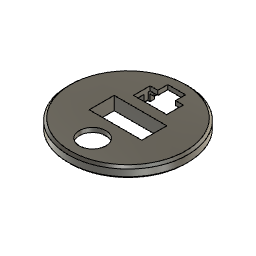
PowerBank RedBull (Autodesk Fusion 360 design; units mm, degrees)
Autodesk Fusion 360 part; units mm, degrees
sketch "Boceto1" plane through (0, 0, 0) normal (0, 0, 1) x (1, 0, 0)
  circle A0 centre (0, 0) radius 27
  dimension "d1" = 54
  constraint coincident A0.centre origin
  measures "d1" diameter of A0
extrude "Extruir1" add sketch "Boceto1" along normal blind 5
sketch "Boceto2" plane through (0, 0, 0) normal (0, 0, -1) x (1, 0, 0)
  circle A0 centre (0, 0) radius 27
  circle A1 centre (0, 0) radius 26
  dimension "d6" = 52
  constraint coincident A0.centre A1.centre
  measures "d6" diameter of A1
extrude "Extruir2" cut sketch "Boceto2" against normal blind 3 contours A1
sketch "Boceto3" plane through (0, 0, 5) normal (0, 0, 1) x (-1, 0, 0)
  circle A0 centre (0, 0) radius 27
  line L0 (-11.4, 5.15) -> (11.4, 5.15)
  line L1 (11.4, 5.15) -> (11.4, -5.15)
  line L2 (11.4, -5.15) -> (-11.4, -5.15)
  line L3 (-11.4, -5.15) -> (-11.4, 5.15)
  line L4 (-11.4, 5.15) -> (11.4, -5.15) construction
  line L5 (11.4, 5.15) -> (-11.4, -5.15) construction
  line L6 (0, -27) -> (0, 27) construction
  line L7 (0, 5.15) -> (0, 16) construction
  circle A1 centre (0, 16) radius 6
  dimension "d9" = 10.3
  dimension "d10" = 22.8
  dimension "d11" = 12
  constraint horizontal L0
  constraint perpendicular L0 L1
  constraint parallel L0 L2
  constraint parallel L1 L3
  constraint coincident L4 A0.centre
  constraint coincident L5 A0.centre
  constraint coincident A0.centre origin
  constraint coincident A0 L6.start
  constraint coincident A0 L6.end
  constraint perpendicular L0 L6
  constraint midpoint L0 L7.start
  constraint coincident L6 L7.end
  constraint perpendicular L0 L7
  constraint coincident L7.end A1.centre
  measures "d9" distance of L0.start L2.end
  measures "d10" distance of L0.start L0.end
  measures "d11" diameter of A1
extrude "Extruir3" cut sketch "Boceto3" against normal blind 3 contours L0 L1 L2 L3 | A1
sketch "Boceto4" plane through (0, 0, 3) normal (0, 0, -1) x (1, 0, 0)
  circle A0 centre (0, 16) radius 6
  line L0 (-11.4, -5.15) -> (-11.4, 5.15)
  line L1 (-11.4, 5.15) -> (11.4, 5.15)
  line L2 (11.4, 5.15) -> (11.4, -5.15)
  line L3 (11.4, -5.15) -> (-11.4, -5.15)
  circle A1 centre (0, 0) radius 26
  line L4 (-12.4, 6.15) -> (12.4, 6.15)
  line L5 (12.4, 6.15) -> (12.4, -6.15)
  line L6 (12.4, -6.15) -> (-12.4, -6.15)
  line L7 (-12.4, -6.15) -> (-12.4, 6.15)
  line L8 (-12.4, 6.15) -> (12.4, -6.15) construction
  line L9 (12.4, 6.15) -> (-12.4, -6.15) construction
  dimension "d14" = 24.8
  dimension "d15" = 12.3
  constraint horizontal L4
  constraint perpendicular L4 L5
  constraint parallel L4 L6
  constraint parallel L5 L7
  constraint coincident L8 A1.centre
  constraint coincident L9 A1.centre
  constraint coincident A1.centre origin
  measures "d14" distance of L5.end L6.end
  measures "d15" distance of L4.end L5.end
extrude "Extruir4" add sketch "Boceto4" along normal blind 4 contours L4 L5 L6 L7
chamfer "Chaflán1" distance 1 angle 45 1 edges at (-25.1728, -9.7636, 5)
extrude "Extruir5" add 1 faces at (12.4, -2.05, 0.3333) along direction (1, 0, 0) blind 5
extrude "Extruir6" add 1 faces at (-12.4, 2.05, 0.3333) along direction (-1, 0, 0) blind 5
extrude "Extruir7" add 1 faces at (17.4, -2.05, 0.3333) along direction (1, 0, 0) blind 1
extrude "Extruir8" add 1 faces at (-17.4, 2.05, 0.3333) along direction (-1, 0, 0) blind 1
chamfer "Chaflán2" distance 1 angle 45 1 edges at (-25.1728, -9.7636, 0)
sketch "Boceto5" plane through (0, 0, 5) normal (0, 0, 1) x (-1, 0, 0)
  line L0 (11.4, 5.15) -> (11.4, -5.15)
  line L1 (11.4, -5.15) -> (-11.4, -5.15)
  line L2 (-11.4, -5.15) -> (-11.4, 5.15)
  line L3 (-11.4, 5.15) -> (11.4, 5.15)
  circle A0 centre (0, 16) radius 6
  circle A1 centre (0, 0) radius 26
  line L4 (0, 0) -> (0, -16)
  line L5 (7.5, -10) -> (-7.5, -10)
  line L6 (-7.5, -10) -> (-7.5, -22)
  line L7 (-7.5, -22) -> (7.5, -22)
  line L8 (7.5, -22) -> (7.5, -10)
  line L9 (7.5, -10) -> (-7.5, -22) construction
  line L10 (-7.5, -10) -> (7.5, -22) construction
  line L11 (-7.5, -10) -> (-7.5, -17.5)
  line L12 (-7.5, -17.5) -> (7.5, -17.5)
  line L13 (0, -17.5) -> (-4, -17.5)
  line L14 (-4, -17.5) -> (-4, -22)
  line L15 (-4, -22) -> (4, -22)
  line L16 (4, -22) -> (4, -17.5)
  point P0 (0, -16)
  dimension "d28" = 16
  dimension "d29" = 15
  dimension "d30" = 12
  dimension "d31" = 7.5
  constraint coincident A1.centre L4.start
  constraint perpendicular L1 L4
  constraint horizontal L5
  constraint perpendicular L5 L6
  constraint parallel L5 L7
  constraint parallel L6 L8
  constraint coincident L9 P0
  constraint coincident L10 P0
  constraint coincident P0 L4.end
  constraint perpendicular L5 L11
  constraint coincident L8 L12.end
  constraint perpendicular L8 L12
  constraint midpoint L12 L13.start
  constraint coincident L12 L13.end
  constraint coincident L7 L14.end
  constraint perpendicular L7 L14
  constraint coincident L7 L15.end
  constraint coincident L12 L16.end
  constraint perpendicular L12 L16
  measures "d28" distance of A1.centre P0
  measures "d29" distance of L6.end L7.end
  measures "d30" distance of L5.end L6.end
  measures "d31" distance of L5.end L11.end
extrude "Extruir9" cut sketch "Boceto5" against normal blind 2 contours L5 L6 L8 L11 L12 L13 | L7 L12 L13 L14 L15 L16
sketch "Boceto6" plane through (0, 0, 3) normal (0, 0, -1) x (1, 0, 0)
  line L0 (-4, -17.5) -> (-7.5, -17.5)
  line L1 (-7.5, -17.5) -> (-7.5, -10)
  line L2 (-7.5, -10) -> (7.5, -10)
  line L3 (7.5, -10) -> (7.5, -17.5)
  line L4 (7.5, -17.5) -> (4, -17.5)
  line L5 (4, -17.5) -> (4, -22)
  line L6 (4, -22) -> (-4, -22)
  line L7 (-4, -22) -> (-4, -17.5)
  line L8 (-18.4, 6.15) -> (18.4, 6.15)
  line L9 (18.4, 6.15) -> (18.4, -6.15)
  line L10 (18.4, -6.15) -> (-18.4, -6.15)
  line L11 (-18.4, -6.15) -> (-18.4, 6.15)
  circle A0 centre (0, 16) radius 6
  circle A1 centre (0, 0) radius 26
  line L12 (4, -22) -> (4, -19)
  line L13 (0, -19) -> (10, -19)
  line L14 (10.3, -19.3) -> (10.3, -16.7)
  line L15 (-10.3, -16.7) -> (10.3, -16.7)
  line L16 (-10.3, -19.3) -> (-10.3, -16.7)
  line L17 (10.3, -19.3) -> (-10.3, -19.3)
  line L18 (12.3, -21.3) -> (12.3, -14.7)
  line L19 (-12.3, -14.7) -> (12.3, -14.7)
  line L20 (-12.3, -21.3) -> (-12.3, -14.7)
  line L21 (12.3, -21.3) -> (-12.3, -21.3)
  dimension "d35" = -2
  constraint coincident L5.end L6.start
  constraint coincident L5 L12.end
  constraint perpendicular L6 L12
  constraint perpendicular L5 L13
extrude "Extruir10" add sketch "Boceto6" along normal blind 3 contours L1 L7 L15 L16 L17 L19 L20 L21 | L3 L5 L12 L14 L15 L17 L18 L19 L21
sketch "Boceto7" plane through (0, 0, 0) normal (0, 0, -1) x (1, 0, 0)
  line L0 (7.5, -14.7) -> (7.5, -16.7)
  line L1 (7.5, -16.7) -> (10.3, -16.7)
  line L2 (10.3, -16.7) -> (10.3, -19.3)
  line L3 (10.3, -19.3) -> (4, -19.3)
  line L4 (4, -19.3) -> (4, -21.3)
  line L5 (4, -21.3) -> (12.3, -21.3)
  line L6 (12.3, -21.3) -> (12.3, -14.7)
  line L7 (12.3, -14.7) -> (7.5, -14.7)
  line L8 (4, -19.3) -> (7.5002, -19.3)
  line L9 (7.5002, -19.3) -> (7.5002, -21.3)
  line L10 (7.5002, -21.3) -> (4, -21.3)
  line L11 (4, -21.3) -> (4, -19.3)
  constraint horizontal L8
  constraint vertical L9
  constraint horizontal L10
  constraint vertical L11
  constraint coincident L5 L9.end
  constraint coincident L3.end L4.start
extrude "Extruir11" cut sketch "Boceto7" against normal blind 3 contours L3 L4 L5 L8 L9 L10 L11
sketch "Boceto8" plane through (0, 0, 0) normal (0, 0, -1) x (1, 0, 0)
  line L0 (-12.3, -21.3) -> (-4, -21.3)
  line L1 (-4, -21.3) -> (-4, -19.3)
  line L2 (-4, -19.3) -> (-10.3, -19.3)
  line L3 (-10.3, -19.3) -> (-10.3, -16.7)
  line L4 (-10.3, -16.7) -> (-7.5, -16.7)
  line L5 (-7.5, -16.7) -> (-7.5, -14.7)
  line L6 (-7.5, -14.7) -> (-12.3, -14.7)
  line L7 (-12.3, -14.7) -> (-12.3, -21.3)
  line L8 (-4, -21.3) -> (-7.5, -21.3)
  line L9 (-7.5, -21.3) -> (-7.5, -19.3)
  line L10 (-7.5, -19.3) -> (-4, -19.3)
  line L11 (-4, -19.3) -> (-4, -21.3)
  line L12 (-12.3, -14.7) -> (-10.3, -14.7)
  line L13 (-10.3, -14.7) -> (-10.3, -21.3)
  line L14 (-10.3, -21.3) -> (-12.3, -21.3)
  line L15 (-12.3, -21.3) -> (-12.3, -14.7)
  line L16 (-10.3, -14.7) -> (-9.3, -14.7)
  line L17 (-9.3, -14.7) -> (-9.3, -16.7)
  line L18 (-9.3, -16.7) -> (-10.3, -16.7)
  line L19 (-10.3, -16.7) -> (-10.3, -14.7)
  line L20 (-10.3, -21.3) -> (-9.3, -21.3)
  line L21 (-9.3, -21.3) -> (-9.3, -19.3)
  line L22 (-9.3, -19.3) -> (-10.3, -19.3)
  line L23 (-10.3, -19.3) -> (-10.3, -21.3)
  dimension "d42" = 1
  dimension "d43" = 1
  constraint horizontal L8
  constraint vertical L9
  constraint horizontal L10
  constraint vertical L11
  constraint coincident L2 L9.end
  constraint coincident L0.end L1.start
  constraint horizontal L12
  constraint vertical L13
  constraint horizontal L14
  constraint vertical L15
  constraint coincident L0 L13.end
  constraint coincident L6.end L7.start
  constraint horizontal L16
  constraint vertical L17
  constraint horizontal L18
  constraint vertical L19
  constraint horizontal L20
  constraint vertical L21
  constraint horizontal L22
  constraint vertical L23
  measures "d42" distance of L12.end L16.end
  measures "d43" distance of L13.end L20.end
extrude "Extruir12" cut sketch "Boceto8" against normal blind 3 contours L0 L1 L2 L8 L9 L10 L11
extrude "Extruir14" add sketch "Boceto8" along normal blind 3 contours L0 L3 L6 L7 L12 L13 L14 L15 L19 L23 | L0 L2 L13 L20 L21 L22 L23 | L4 L6 L13 L16 L17 L18 L19
sketch "Boceto9" plane through (0, 0, 0) normal (0, 0, -1) x (1, 0, 0)
  line L0 (7.5002, -19.3) -> (7.5002, -21.3)
  line L1 (7.5002, -21.3) -> (12.3, -21.3)
  line L2 (12.3, -21.3) -> (12.3, -14.7)
  line L3 (12.3, -14.7) -> (7.5, -14.7)
  line L4 (7.5, -14.7) -> (7.5, -16.7)
  line L5 (7.5, -16.7) -> (10.3, -16.7)
  line L6 (10.3, -16.7) -> (10.3, -19.3)
  line L7 (10.3, -19.3) -> (7.5002, -19.3)
  line L8 (12.3, -14.7) -> (9.3, -14.7)
  line L9 (9.3, -14.7) -> (9.3, -16.7)
  line L10 (9.3, -16.7) -> (12.3, -16.7)
  line L11 (12.3, -16.7) -> (12.3, -14.7)
  line L12 (12.3, -21.3) -> (9.3, -21.3)
  line L13 (9.3, -21.3) -> (9.3, -19.3)
  line L14 (9.3, -19.3) -> (12.3, -19.3)
  line L15 (12.3, -19.3) -> (12.3, -21.3)
  dimension "d48" = 3
  dimension "d49" = 3
  constraint horizontal L8
  constraint vertical L9
  constraint horizontal L10
  constraint vertical L11
  constraint coincident L2.end L3.start
  constraint horizontal L12
  constraint vertical L13
  constraint horizontal L14
  constraint vertical L15
  constraint coincident L1.end L2.start
  measures "d48" distance of L2.end L8.end
  measures "d49" distance of L1.end L12.end
extrude "Extruir15" add sketch "Boceto9" along normal blind 3 contours L1 L2 L7 L12 L13 L14 L15 | L2 L6 L10 L14 | L2 L3 L5 L8 L9 L10 L11
sketch "Boceto10" plane through (0, 0, -1) normal (0, 0, -1) x (1, 0, 0)
  line L0 (11.4, 5.15) -> (11.4, -5.15)
  line L1 (11.4, -5.15) -> (-11.4, -5.15)
  line L2 (-11.4, -5.15) -> (-11.4, 5.15)
  line L3 (-11.4, 5.15) -> (11.4, 5.15)
  line L4 (-18.4, -6.15) -> (18.4, -6.15)
  line L5 (18.4, -6.15) -> (18.4, 6.15)
  line L6 (18.4, 6.15) -> (-18.4, 6.15)
  line L7 (-18.4, 6.15) -> (-18.4, -6.15)
  line L8 (-11.4, 5.15) -> (-16.4, 5.15)
  line L9 (-16.4, 5.15) -> (-16.4, -5.15)
  line L10 (-16.4, -5.15) -> (-11.4, -5.15)
  line L11 (-11.4, -5.15) -> (-11.4, 5.15)
  line L12 (11.4, 5.15) -> (16.4, 5.15)
  line L13 (16.4, 5.15) -> (16.4, -5.15)
  line L14 (16.4, -5.15) -> (11.4, -5.15)
  line L15 (11.4, -5.15) -> (11.4, 5.15)
  circle A0 centre (-13.9, 0) radius 1.5
  circle A1 centre (13.9, 0) radius 1.5
  dimension "d52" = 5
  dimension "d53" = 5
  dimension "d54" = 3
  dimension "d55" = 3
  constraint horizontal L8
  constraint vertical L9
  constraint horizontal L10
  constraint vertical L11
  constraint coincident L2.end L3.start
  constraint horizontal L12
  constraint vertical L13
  constraint horizontal L14
  constraint vertical L15
  constraint coincident L0.start L3.end
  measures "d52" distance of L2.end L8.end
  measures "d53" distance of L0.start L12.end
  measures "d54" diameter of A0
  measures "d55" diameter of A1
extrude "Extruir16" cut sketch "Boceto10" against normal blind 4 contours A0 | A1
thread "Rosca1" "ISO Metric profile 3.0 M3x0.5 6H" major diameter 3.086 minor diameter 2.529 pitch 0.5 angle 60 resizes the face on face at (15.3925, 0.1494, 0.3333)
thread "Rosca2" "ISO Metric profile 3.0 M3x0.5 6H" major diameter 3.086 minor diameter 2.529 pitch 0.5 angle 60 resizes the face on face at (-12.4019, 0.0748, 1.6667)
sketch "Boceto11" plane through (0, 0, 5) normal (0, 0, 1) x (-1, 0, 0)
  line L0 (7.5, -17.5) -> (4, -17.5)
  line L1 (4, -17.5) -> (4, -22)
  line L2 (4, -22) -> (-4, -22)
  line L3 (-4, -22) -> (-4, -17.5)
  line L4 (-4, -17.5) -> (-7.5, -17.5)
  line L5 (-7.5, -17.5) -> (-7.5, -10)
  line L6 (-7.5, -10) -> (7.5, -10)
  line L7 (7.5, -10) -> (7.5, -17.5)
  line L8 (11.4, 5.15) -> (11.4, -5.15)
  line L9 (11.4, -5.15) -> (-11.4, -5.15)
  line L10 (-11.4, -5.15) -> (-11.4, 5.15)
  line L11 (-11.4, 5.15) -> (11.4, 5.15)
  circle A0 centre (0, 16) radius 6
  circle A1 centre (0, 0) radius 26
  line L12 (11.9, -5.65) -> (-11.9, -5.65)
  line L13 (-11.9, -5.65) -> (-11.9, 5.65)
  line L14 (-11.9, 5.65) -> (11.9, 5.65)
  line L15 (11.9, 5.65) -> (11.9, -5.65)
  dimension "d58" = -0.5
extrude "Extruir17" cut sketch "Boceto11" against normal blind 10 contours L12 L13 L14 L15
extrude "Extruir13" [suppressed]
equation "d1 = Dex"
equation "Dex = 54 mm"
equation "Din = 52 mm"
equation "d6 = Din"
